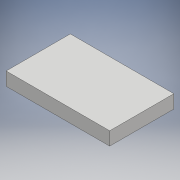
# Autodesk Inventor part: wall
Saved by Autodesk Inventor 2017 (Build 210142000, 142)
## iProperties
Created: 2017-10-30
Part Number: wall
Material: Generic
Document SubType Name: Modeling
Designer: DesignPC02
Density: 1 g/cm^3
Appearance: Default
Author: DesignPC02
Autodesk Inventor part; units mm, degrees
ref_plane "YZ Plane" through (0, 0, 0) normal (1, 0, 0) x (0, 1, 0)
ref_plane "XZ Plane" through (0, 0, 0) normal (0, 1, 0) x (-1, 0, 0)
ref_plane "XY Plane" through (0, 0, 0) normal (0, 0, 1) x (1, 0, 0)
sketch "Sketch1" plane through (0, 0, 0) normal (0, 0, 1) x (1, 0, 0)
  line L0 (-2340, -1450) -> (2340, -1450)
  line L1 (2340, -1450) -> (2340, 1450)
  line L2 (2340, 1450) -> (-2340, 1450)
  line L3 (-2340, 1450) -> (-2340, -1450)
  line L4 (-2340, -1450) -> (2340, 1450) construction
  line L5 (2340, -1450) -> (-2340, 1450) construction
  point P0 (0, 0)
  dimension "d0" = 4680
  dimension "d1" = 2900
  constraints: 12 end point, 2 midpoint, 2 parallel, 1 horizontal, 1 perpendicular
  measures "d0" distance of L2.end L1.end
  measures "d1" distance of L1.end L0.end
extrude "Extrusion1" add sketch "Sketch1" along normal blind 600
body "Solid1"
